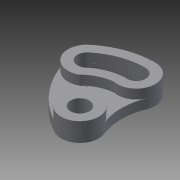
# Autodesk Inventor part: 4-1
Saved by Autodesk Inventor 2015 SP2 (Build 190223200, 223)
## iProperties
Created: 2015-09-16
Part Number: 4-1
Material: Generic
Document SubType Name: Modeling
Designer: Brandon
Density: 1 g/cm^3
Appearance: Default
Author: Brandon
Autodesk Inventor part; units mm, degrees
ref_plane "YZ Plane" through (0, 0, 0) normal (1, 0, 0) x (0, 1, 0)
ref_plane "XZ Plane" through (0, 0, 0) normal (0, 1, 0) x (-1, 0, 0)
ref_plane "XY Plane" through (0, 0, 0) normal (0, 0, 1) x (1, 0, 0)
sketch "Sketch1" plane through (0, 0, 0) normal (0, 1, 0) x (-1, 0, 0)
  circle A0 centre (0, 0) radius 12.7
  circle A1 centre (0, 0) radius 25.4
  arc A2 (0.6057, -63.5145) -> (2.1044, -88.7244) centre (0, -76.2) ccw
  arc A3 (55.4189, -69.3196) -> (40.3623, -49.0442) centre (48.9804, -58.3726) ccw
  arc A4 (0, -88.7494) -> (55.4189, -69.3196) centre (0, 0) ccw
  arc A5 (0, -63.5173) -> (40.3623, -49.0442) centre (0, 0) ccw
  arc A6 (3.9125, -51.1031) -> (2.4005, -101.4863) centre (0, -76.2) ccw
  arc A7 (63.3952, -79.286) -> (29.8513, -41.6622) centre (48.9804, -58.3726) ccw
  arc A8 (0, -101.5147) -> (67.073, -76.2) centre (0, 0) ccw
  arc A9 (0, -51.2527) -> (35.8456, -36.6324) centre (0, 0) ccw
  arc A10 (73.1376, -50.5246) -> (11.9236, 22.4274) centre (-47.7394, -89.7941) ccw
  arc A11 (-23.5464, -66.675) -> (-23.5464, -9.525) centre (-94.1857, -38.1) ccw
  dimension "d0" = 25.4
  dimension "d1" = 50.8
  dimension "d5" = 25.4
  dimension "d6" = 25.4
  dimension "d7" = 50.8
  dimension "d8" = 50.8
  constraints: 32 point on circle, 12 centre point, 8 coincident, 4 tangent
  measures "d0" diameter of A0
  measures "d1" diameter of A1
  measures "d5" diameter of A2
  measures "d6" diameter of A3
  measures "d7" diameter of A6
  measures "d8" diameter of A7
extrude "Extrusion1" add sketch "Sketch1" along normal blind 12.7 contours A1 | A1 A10 A7 A9 A6 A11 | A7 A8 A6 A9
sketch "Sketch2" plane through (0, 12.7, 0) normal (0, 1, 0) x (1, 0, 0)
  circle A0 centre (0, 0) radius 12.7
  circle A1 centre (0, 0) radius 25.4
  arc A2 (-56.6694, 68.4805) -> (-39.457, 49.9705) centre (-48.9804, 58.3726) ccw
  arc A3 (-63.3952, 79.286) -> (-29.0277, 42.6547) centre (-48.9804, 58.3726) ccw
  arc A4 (-1.8946, 63.6421) -> (-0.6072, 88.8855) centre (0, 76.2) ccw
  arc A5 (-5.1814, 51.3341) -> (-2.4005, 101.4863) centre (0, 76.2) ccw
  arc A6 (-2.4005, 101.4863) -> (-67.073, 76.2) centre (0, 0) ccw
  arc A7 (0, 51.5949) -> (-36.9661, 35.9937) centre (0, 0) ccw
  arc A8 (-0.6072, 63.6674) -> (-42.3597, 47.5349) centre (0, 0) ccw
  arc A9 (-0.6072, 88.8855) -> (-58.1288, 67.2461) centre (0, 0) ccw
  dimension "d16" = 25.4
  dimension "d17" = 50.8
  dimension "d21" = 25.4
  dimension "d22" = 50.8
  dimension "d23" = 25.4
  dimension "d24" = 50.8
  constraints: 25 point on circle, 10 centre point, 8 coincident
  measures "d16" diameter of A0
  measures "d17" diameter of A1
  measures "d21" diameter of A2
  measures "d22" diameter of A3
  measures "d23" diameter of A4
  measures "d24" diameter of A5
extrude "Extrusion2" add sketch "Sketch2" along normal blind 12.7 contours A1 | A6 A5 A7 A3
body "Solid1"
